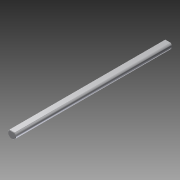
# Autodesk Inventor part: 10-0080
Saved by Autodesk Inventor 2015 SP1 (Build 190203100, 203)
## iProperties
Category: Axle Kit
Company: Autodesk Inc.
Created: 2014-11-30
Part Number: 10-0080
Material: Aluminum 6061
Document SubType Name: Modeling
Designer: Matrix
Density: 2.7 g/cm^3
Appearance: Aluminum - Polished
Catalog Web Link: http://matrixrobotics.com/
Vendor: Matrix
Author: Autodesk Inc.
Autodesk Inventor part; units mm, degrees
ref_plane "YZ Plane" through (0, 0, 0) normal (1, 0, 0) x (0, 1, 0)
ref_plane "XZ Plane" through (0, 0, 0) normal (0, 1, 0) x (-1, 0, 0)
ref_plane "XY Plane" through (0, 0, 0) normal (0, 0, 1) x (1, 0, 0)
sketch "Sketch1" plane through (0, 0, 0) normal (0, 1, 0) x (-1, 0, 0)
  circle A0 centre (0, 0) radius 2
  dimension "d0" = 4
  constraints: 1 centre point, 1 coincident
  measures "d0" diameter of A0
extrude "Extrusion1" add sketch "Sketch1" against normal blind 80
sketch "Sketch2" plane through (0, -80, 0) normal (0, -1, 0) x (1, 0, 0)
  circle A0 centre (0, 0) radius 2 projected
  line L0 (-1.3229, 1.5) -> (1.3229, 1.5)
  circle A1 centre (0, 0) radius 2 projected
  dimension "d3" = 0.5
  constraints: 2 end point, 2 point on circle, 1 horizontal, 2 other
  measures "d3" distance edge to line of A0 L0
extrude "Extrusion2" cut sketch "Sketch2" against normal through all contours L0 A0 picked at (-0.3089, 1.5908)
chamfer "Chamfer1" distance 0.2 angle 45 4 edges at (0, -80, -2) (0, -80, 1.5) (0, 0, -2) (0, 0, 1.5)
body "Solid1"
